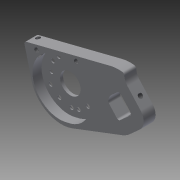
# Autodesk Inventor part: mountthatshopefullyslightlyeasiertomachine
Saved by Autodesk Inventor 2014 SP1 (Build 180222100, 222)
## iProperties
Created: 2014-05-15
Part Number: mountthatshopefullyslightlyeasiertomachine
Material: Generic
Document SubType Name: Modeling
Designer: brent
Density: 1 g/cm^3
Appearance: Default
Author: brent
Autodesk Inventor part; units mm, degrees
ref_plane "YZ Plane" through (0, 0, 0) normal (1, 0, 0) x (0, 1, 0)
ref_plane "XZ Plane" through (0, 0, 0) normal (0, 1, 0) x (-1, 0, 0)
ref_plane "XY Plane" through (0, 0, 0) normal (0, 0, 1) x (1, 0, 0)
derived "mountsketch_alt.ipt"
sketch "Sketch1" plane through (0, 0, 0) normal (0, 0, 1) x (1, 0, 0)
  circle A0 centre (-34.7277, 175.7429) radius 11 projected
  circle A1 centre (-53.3698, 187.425) radius 2.15 projected
  circle A2 centre (-34.7277, 175.7429) radius 33 projected
  circle A3 centre (-46.4099, 157.1008) radius 2.15 projected
  circle A4 centre (-16.0856, 164.0607) radius 2.15 projected
  circle A5 centre (-23.0456, 194.3849) radius 2.15 projected
  line L0 (127, 127.3759) -> (61.9125, 127.3759) projected
  line L1 (-105.8581, 0) -> (165.8097, 0) projected
  line L2 (33.0604, 216.3483) -> (58.3844, 188.2233) projected
  line L3 (58.3844, 188.2233) -> (34.6008, 166.8084) projected
  line L4 (-23.0456, 194.3849) -> (-16.0856, 164.0607) projected
  line L5 (-34.7277, 175.7429) -> (26.1158, 189.7076) projected
  line L6 (26.1158, 189.7076) -> (-32.871, 176.169) projected
  circle A6 centre (-10.8773, 175.6436) radius 2.15 projected
  line L7 (26.1158, 189.7076) -> (-36.5845, 175.3167) projected
  circle A7 centre (-25.9478, 156.059) radius 2.15 projected
  circle A8 centre (-32.3456, 198.1627) radius 2.15 projected
  circle A9 centre (-54.8647, 176.6944) radius 2.15 projected
  circle A10 centre (-33.3964, 154.1753) radius 2.15 projected
  circle A11 centre (-17.3267, 185.9534) radius 2.15 projected
  circle A12 centre (-47.2211, 194.5745) radius 2.15 projected
  circle A13 centre (-55.8422, 164.68) radius 2.15 projected
  line L8 (16.1602, 187.2887) -> (24.9131, 177.5677) projected
  line L9 (25.6305, 177.5301) -> (38.2774, 188.9173) projected
  line L10 (38.315, 189.6348) -> (29.5621, 199.3558) projected
  line L11 (33.0604, 216.3483) -> (-38.3131, 208.5475) projected
  line L12 (34.6008, 166.8084) -> (-22.9948, 144.8991) projected
  circle A14 centre (26.1158, 189.7076) radius 34.33 projected
  line L13 (33.0604, 216.3483) -> (32.281, 223.4794) projected
  line L14 (27.0217, 204.0752) -> (40.4485, 189.1632) projected
  line L15 (16.1602, 187.2887) -> (26.1028, 176.2463) projected
  line L16 (26.1028, 176.2463) -> (40.4485, 189.1632) projected
  line L17 (27.0217, 204.0752) -> (19.3412, 197.1596) projected
  ellipse E0 centre (22.8611, 193.3223) end of major axis (29.5621, 199.3558) minor radius 5.2071 (19.3412, 197.1596) -> (16.1602, 187.2887) ccw projected
  line L18 (-42.7935, 207.742) -> (17.725, 222.9963) projected
  line L19 (-42.7935, 207.742) -> (-74.7926, 199.6762) projected
  line L20 (-74.7926, 199.6762) -> (-66.7269, 167.6771) projected
  point P0 (0, 0)
  point P1 (-2.1526, 151.7421)
  point P2 (-7.3054, 194.1009)
  point P3 (0.7264, 212.8144)
  constraints: 4 other
extrude "Extrusion11" add sketch "Sketch1" along normal blind 12.7 contours A2 A14 | L11 A14 A2 | A2 L18 A14 L11 | A2 L20 L19 | A14 L11 L2 L3 L12 A2 | A2 L5 A14 | A14 L13 L11 | A2 A14 L5 | A2 A14 L12
fillet "Fillet7" radius 25.4 1 edges at (34.6008, 166.8084, 6.35)
fillet "Fillet7" radius 2.54 1 edges at (32.281, 223.4794, 6.35)
fillet "Fillet7" radius 12.7 2 edges at (58.3844, 188.2233, 6.35) (33.0604, 216.3483, 6.35)
sketch "Sketch17" plane through (-34.7277, 175.7429, 12.7) normal (0, 0, 1) x (0.4619488, 0.8869066, 0)
  circle A0 centre (10.9297, -21.199) radius 2.15 projected
  circle A1 centre (0, 0) radius 11 projected
  circle A2 centre (-13.4019, -16.88) radius 2.15 projected
  circle A3 centre (-19.5655, 13.6161) radius 2.15 projected
  circle A4 centre (10.9306, 19.7797) radius 2.15 projected
  circle A5 centre (17.0942, -10.7163) radius 2.15 projected
  circle A6 centre (-18.5134, -11.1439) radius 2.15 projected
  circle A7 centre (-8.4583, 18.2992) radius 2.15 projected
  circle A8 centre (20.9848, 8.2441) radius 2.15 projected
  circle A9 centre (21.9303, -1.7493) radius 2.15 projected
  circle A10 centre (-1.7493, -21.9303) radius 2.15 projected
  circle A11 centre (-21.9303, 1.7493) radius 2.15 projected
  circle A12 centre (1.7493, 21.9303) radius 2.15 projected
  arc A13 (-22.024, -18.7701) -> (22.024, 18.7701) centre (1.2357, -1.4499) ccw
  arc A14 (22.024, 18.7701) -> (-22.024, -18.7701) centre (-1.2357, 1.4499) ccw
  line L0 (-20.836, -20.2606) -> (-23.3073, -17.3608)
  line L1 (23.3073, 17.3608) -> (20.836, 20.2606)
  point P0 (65.9055, 28.4481)
  point P1 (29.8536, 27.856)
  point P2 (5.2355, 34.1004)
  point P3 (-139.8251, -111.9844)
  point P4 (3.0016, 34.3692)
  dimension "d178" = 58
  dimension "d179" = 58
  constraints: 8 point on circle, 4 end point, 4 tangent, 2 centre point, 2 coincident
  measures "d178" diameter of A14
  measures "d179" diameter of A13
sketch "Sketch12" plane through (49.8864, 197.6612, 12.7) normal (0.7431448, 0.6691306, 0) x (0, 0, -1)
  line L0 (12.7, 0) -> (12.7, 21.0486) projected
  line L1 (12.7, 13.589) -> (12.7, 0) projected
  line L2 (12.7, 13.589) -> (0, 13.589) projected
  line L3 (0, 0) -> (0, 13.589) projected
  line L4 (12.7, 0) -> (0, 0) projected
  circle A0 centre (6.35, 9.779) radius 2.413
  line L5 (12.7, 14.859) -> (12.7, 0) projected
  line L6 (12.7, 14.859) -> (0, 14.859) projected
  line L7 (0, 0) -> (0, 14.859) projected
  line L8 (12.7, 0) -> (0, 0) projected
  point P0 (12.7, -113.5104)
  dimension "d99" = 4.826
  dimension "d122" = 6.35
  dimension "d123" = 5.08
  constraints: 1 centre point
  measures "d99" diameter of A0
  measures "d122" distance from line of L0 A0.centre
  measures "d123" distance from line of L6 A0.centre
sketch "Sketch13" plane through (48.9464, 179.7253, 0) normal (0.6691306, -0.7431448, 0) x (0.7431448, 0.6691306, 0)
  line L0 (-14.5567, 12.7) -> (0, 12.7) projected
  line L1 (-18.034, 0) -> (0, 0) projected
  line L2 (-18.034, 0) -> (-18.034, 12.7) projected
  line L3 (0, 12.7) -> (-18.034, 12.7) projected
  line L4 (0, 0) -> (0, 12.7) projected
  circle A0 centre (-9.017, 6.35) radius 2.413
  point P0 (-156.634, 0)
  dimension "d100" = 4.826
  dimension "d101" = 9.017
  dimension "d102" = 6.35
  constraints: 1 centre point
  measures "d100" diameter of A0
  measures "d101" distance from line of A0.centre L4
  measures "d102" distance from line of A0.centre L0
extrude "Extrusion13" cut sketch "Sketch13" against normal blind 25.4 contours A0
extrude "Extrusion14" cut sketch "Sketch12" against normal blind 25.4 contours A0
thread "Thread5" size "10-32 UNF" class "2B" standard "ANSI Unified Screw Threads" full length
thread "Thread6" size "10-32 UNF" class "2B" standard "ANSI Unified Screw Threads" full length
sketch "Sketch16" plane through (-34.7277, 175.7429, 0) normal (0, 0, -1) x (-0.4619488, -0.8869066, 0)
  line L0 (-38.0971, 0.9443) -> (-44.0427, -11.275) projected
  line L1 (-44.0427, -11.275) -> (-60.259, -3.3847) projected
  line L2 (-60.259, -3.3847) -> (-54.3134, 8.8346) projected
  arc A0 (-65.8938, -45.2024) -> (-65.8938, -45.2024) centre (-77.7906, -49.6473) ccw projected
  line L3 (-58.5269, -64.9197) -> (-65.8938, -45.2024) projected
  arc A1 (-58.5269, -64.9197) -> (-42.1852, -72.3715) centre (-46.6302, -60.4747) ccw projected
  line L4 (-28.5493, -67.2767) -> (-42.1852, -72.3715) projected
  arc A2 (-28.5493, -67.2767) -> (-20.5555, -62.4595) centre (-37.4392, -43.4832) ccw projected
  line L5 (21.9355, -24.6543) -> (-20.5555, -62.4595) projected
  arc A3 (21.9355, -24.6543) -> (21.9355, 24.6543) centre (0, 0) ccw projected
  line L6 (-34.7521, 29.5687) -> (-5.2355, 34.1004) projected
  circle A4 centre (-1.7493, 21.9303) radius 2.15 projected
  circle A5 centre (21.9303, 1.7493) radius 2.15 projected
  circle A6 centre (1.7493, -21.9303) radius 2.15 projected
  circle A7 centre (-21.9303, -1.7493) radius 2.15 projected
  circle A8 centre (-20.9848, 8.2441) radius 2.15 projected
  circle A9 centre (8.4583, 18.2992) radius 2.15 projected
  circle A10 centre (18.5134, -11.1439) radius 2.15 projected
  circle A11 centre (-17.0942, -10.7163) radius 2.15 projected
  circle A12 centre (-10.9306, 19.7797) radius 2.15 projected
  circle A13 centre (19.5655, 13.6161) radius 2.15 projected
  circle A14 centre (13.4019, -16.88) radius 2.15 projected
  circle A15 centre (-10.9297, -21.199) radius 2.15 projected
  circle A16 centre (0, 0) radius 11 projected
  line L7 (-72.1881, 22.3034) -> (-62.1724, -42.9322)
  line L8 (-62.1724, -42.9322) -> (37.6257, -27.6099)
  line L9 (37.6257, -27.6099) -> (27.6099, 37.6257)
  line L10 (27.6099, 37.6257) -> (-72.1881, 22.3034)
  point P0 (-51.5181, 22.1934)
  point P1 (-5.2355, 34.1004)
  point P2 (139.8251, -111.9844)
  point P3 (-29.8536, 27.856)
  point P4 (-65.9055, 28.4481)
  point P5 (-30.9895, -27.5591)
  point P6 (-70.7348, -39.0877)
  point P7 (-3.0016, 34.3692)
  dimension "d117" = 100.9674
  dimension "d118" = 66
  constraints: 8 end point, 2 parallel, 1 perpendicular, 1 tangent, 9 other
  measures "d117" distance between parallel lines of L9 L7
  measures "d118" distance between parallel lines of L10 L8
extrude "Extrusion15" cut sketch "Sketch17" against normal blind 9.525 contours A14 A13
fillet "Fillet8" radius 2.3813 3 edges at (27.0217, 204.0752, 6.35) (40.4485, 189.1632, 6.35) (26.1028, 176.2463, 6.35)
fillet "Fillet9" radius 2.54 1 edges at (-74.7926, 199.6762, 6.35)
sketch "Sketch18" plane through (-34.7277, 175.7429, 0) normal (0, 0, -1) x (-0.4619488, -0.8869066, 0)
  arc A0 (-58.5269, -64.9197) -> (-42.1852, -72.3715) centre (-46.6302, -60.4747) ccw projected
  line L0 (-28.5493, -67.2767) -> (-42.1852, -72.3715) projected
  arc A1 (-28.5493, -67.2767) -> (-20.5555, -62.4595) centre (-37.4392, -43.4832) ccw projected
  line L1 (21.9355, -24.6543) -> (-20.5555, -62.4595) projected
  arc A2 (21.9355, -24.6543) -> (21.9355, 24.6543) centre (0, 0) ccw projected
  line L2 (-34.7521, 29.5687) -> (-5.2355, 34.1004) projected
  arc A3 (-41.8032, 30.5011) -> (-34.7521, 29.5687) centre (-36.6794, 42.1216) ccw projected
  arc A4 (-66.1399, -24.692) -> (-72.6369, -35.4594) centre (-40.492, -47.5116) ccw projected
  arc A5 (-72.6369, -35.4594) -> (-71.6697, -38.463) centre (-70.2585, -36.3511) ccw projected
  line L3 (-70.7348, -39.0877) -> (-71.6697, -38.463) projected
  arc A6 (-65.8938, -45.2024) -> (-65.8938, -45.2024) centre (-77.7906, -49.6473) ccw projected
  line L4 (-58.5269, -64.9197) -> (-65.8938, -45.2024) projected
  circle A7 centre (-1.7493, 21.9303) radius 2.15 projected
  circle A8 centre (21.9303, 1.7493) radius 2.15 projected
  circle A9 centre (1.7493, -21.9303) radius 2.15 projected
  circle A10 centre (-21.9303, -1.7493) radius 2.15 projected
  circle A11 centre (-20.9848, 8.2441) radius 2.15 projected
  circle A12 centre (8.4583, 18.2992) radius 2.15 projected
  circle A13 centre (18.5134, -11.1439) radius 2.15 projected
  circle A14 centre (-17.0942, -10.7163) radius 2.15 projected
  circle A15 centre (-10.9306, 19.7797) radius 2.15 projected
  circle A16 centre (19.5655, 13.6161) radius 2.15 projected
  circle A17 centre (13.4019, -16.88) radius 2.15 projected
  circle A18 centre (0, 0) radius 11 projected
  circle A19 centre (-10.9297, -21.199) radius 2.15 projected
  ellipse E0 centre (-42.1944, -42.9551) end of major axis (-50.6411, -46.111) minor radius 5.2071 (-33.7477, -39.7992) -> (-43.9717, -38.0606) ccw projected
  line L5 (-33.7477, -39.7992) -> (-29.3806, -51.4878) projected
  arc A20 (-30.7778, -54.5518) -> (-29.3806, -51.4878) centre (-31.6112, -52.3212) ccw projected
  line L6 (-30.7778, -54.5518) -> (-44.3995, -59.6413) projected
  arc A21 (-47.4636, -58.2441) -> (-44.3995, -59.6413) centre (-45.233, -57.4107) ccw projected
  line L7 (-47.4636, -58.2441) -> (-52.8198, -43.9085) projected
  arc A22 (-51.4226, -40.8445) -> (-52.8198, -43.9085) centre (-50.5891, -43.0751) ccw projected
  line L8 (-51.4226, -40.8445) -> (-43.9717, -38.0606) projected
  line L9 (-87.4828, -33.6647) -> (-43.6118, -82.9733)
  line L10 (-43.6118, -82.9733) -> (46.5898, -2.7188)
  line L11 (46.5898, -2.7188) -> (2.7188, 46.5898)
  line L12 (2.7188, 46.5898) -> (-87.4828, -33.6647)
  point P0 (139.8251, -111.9844)
  point P1 (-65.4837, -33.2012)
  point P2 (-3.0016, 34.3692)
  dimension "d125" = 66
  dimension "d126" = 120.7357
  constraints: 8 end point, 2 parallel, 1 collinear, 1 perpendicular, 1 tangent, 8 other
  measures "d125" distance between parallel lines of L10 L12
  measures "d126" distance between parallel lines of L11 L9
sketch "Sketch19" plane through (-34.7277, 175.7429, 0) normal (0, 0, -1) x (-0.8869066, 0.4619488, 0)
  arc A0 (44.9014, 0.8211) -> (44.6922, 4.4071) centre (43.0038, 2.5095) ccw projected
  line L0 (-24.692, 66.1399) -> (44.6922, 4.4071) projected
  arc A1 (-24.692, 66.1399) -> (-35.4594, 72.6369) centre (-47.5116, 40.492) ccw projected
  arc A2 (-35.4594, 72.6369) -> (-38.463, 71.6697) centre (-36.3511, 70.2585) ccw projected
  arc A3 (-45.2024, 65.8938) -> (-45.2024, 65.8938) centre (-49.6473, 77.7906) ccw projected
  line L1 (-64.9197, 58.5269) -> (-45.2024, 65.8938) projected
  arc A4 (-64.9197, 58.5269) -> (-72.3715, 42.1852) centre (-60.4747, 46.6302) ccw projected
  line L2 (-67.2767, 28.5493) -> (-72.3715, 42.1852) projected
  arc A5 (-67.2767, 28.5493) -> (-62.4595, 20.5555) centre (-43.4832, 37.4392) ccw projected
  line L3 (-24.6543, -21.9355) -> (-62.4595, 20.5555) projected
  arc A6 (-24.6543, -21.9355) -> (24.6543, -21.9355) centre (0, 0) ccw projected
  line L4 (44.9014, 0.8211) -> (24.6543, -21.9355) projected
  ellipse E0 centre (-42.9551, 42.1944) end of major axis (-46.111, 50.6411) minor radius 5.2071 (-39.7992, 33.7477) -> (-38.0606, 43.9717) ccw projected
  line L5 (-39.7992, 33.7477) -> (-51.4878, 29.3806) projected
  arc A7 (-54.5518, 30.7778) -> (-51.4878, 29.3806) centre (-52.3212, 31.6112) ccw projected
  line L6 (-54.5518, 30.7778) -> (-59.6413, 44.3995) projected
  arc A8 (-58.2441, 47.4636) -> (-59.6413, 44.3995) centre (-57.4107, 45.233) ccw projected
  line L7 (-58.2441, 47.4636) -> (-43.9085, 52.8198) projected
  arc A9 (-40.8445, 51.4226) -> (-43.9085, 52.8198) centre (-43.0751, 50.5891) ccw projected
  line L8 (-40.8445, 51.4226) -> (-38.0606, 43.9717) projected
  circle A10 centre (0, 0) radius 11 projected
  circle A11 centre (-21.199, 10.9297) radius 2.15 projected
  circle A12 centre (-16.88, -13.4019) radius 2.15 projected
  circle A13 centre (13.6161, -19.5655) radius 2.15 projected
  circle A14 centre (19.7797, 10.9306) radius 2.15 projected
  circle A15 centre (-10.7163, 17.0942) radius 2.15 projected
  circle A16 centre (-11.1439, -18.5134) radius 2.15 projected
  circle A17 centre (18.2992, -8.4583) radius 2.15 projected
  circle A18 centre (8.2441, 20.9848) radius 2.15 projected
  circle A19 centre (-1.7493, 21.9303) radius 2.15 projected
  circle A20 centre (-21.9303, -1.7493) radius 2.15 projected
  circle A21 centre (1.7493, -21.9303) radius 2.15 projected
  circle A22 centre (21.9303, 1.7493) radius 2.15 projected
  line L9 (-88.3349, 34.4229) -> (-44.4639, 83.7315)
  line L10 (-44.4639, 83.7315) -> (46.5898, 2.7188)
  line L11 (46.5898, 2.7188) -> (2.7188, -46.5898)
  line L12 (2.7188, -46.5898) -> (-88.3349, 34.4229)
  point P0 (-33.2012, 65.4837)
  point P1 (-111.9844, -139.8251)
  dimension "d128" = 66
  dimension "d129" = 121.8763
  constraints: 8 end point, 3 tangent, 2 parallel, 1 collinear, 1 perpendicular, 1 point on line, 3 other
  measures "d128" distance between parallel lines of L12 L10
  measures "d129" distance between parallel lines of L11 L9
sketch "Sketch21" plane through (17.725, 222.9963, 12.7) normal (-0.2444163, 0.9696704, 0) x (0.9696704, 0.2444163, 0)
  line L0 (0, 12.7) -> (-92.8714, 12.7) projected
  circle A0 centre (-89.0614, 8.89) radius 2.413
  line L1 (-95.4114, 12.7) -> (-95.4114, 0) projected
  point P0 (-71.6914, 12.7)
  dimension "d138" = 4.826
  dimension "d140" = 3.81
  dimension "d167" = 6.35
  constraints: 1 centre point
  measures "d138" diameter of A0
  measures "d140" distance from line of A0.centre L0
  measures "d167" distance from line of L1 A0.centre
extrude "Extrusion17" cut sketch "Sketch21" against normal blind 12.7
thread "Thread7" size "10-32 UNF" class "2B" standard "ANSI Unified Screw Threads" full length
sketch "Sketch22" plane through (-34.7277, 175.7429, 0) normal (0, 0, -1) x (-0.8869066, 0.4619488, 0)
  arc A0 (-24.692, 66.1399) -> (-35.4594, 72.6369) centre (-47.5116, 40.492) ccw projected
  circle A1 centre (0, 0) radius 11 projected
  circle A2 centre (-47.5116, 40.492) radius 31.83
  circle A3 centre (0, 0) radius 11.935
  line L0 (10.2328, 6.1427) -> (-20.2212, 56.8743)
  line L1 (-59.3607, 10.9497) -> (-4.4429, -11.0772)
  circle A4 centre (0, 0) radius 28
  circle A5 centre (1.2967, 36.6425) radius 2.413
  circle A6 centre (33.9359, 7.6026) radius 2.413
  line L2 (0, 0) -> (-47.5116, 40.492)
  line L3 (-24.692, 66.1399) -> (44.6922, 4.4071) projected
  line L4 (44.9014, 0.8211) -> (24.6543, -21.9355) projected
  point P0 (-111.9844, -139.8251)
  dimension "d146" = 63.66
  dimension "d147" = 23.87
  dimension "d148" = 56
  dimension "d149" = 4.826
  dimension "d150" = 4.826
  dimension "d181" = 12.7
  dimension "d182" = 4.7625
  dimension "d184" = 4.7625
  dimension "d185" = 43.688
  constraints: 6 end point, 5 centre point, 4 point on circle, 4 tangent, 3 coincident
  measures "d146" diameter of A2
  measures "d147" diameter of A3
  measures "d148" diameter of A4
  measures "d149" diameter of A5
  measures "d150" diameter of A6
  measures "d181" distance from line of L4 A6.centre
  measures "d182" distance from line of L3 A6.centre
  measures "d184" distance from line of L3 A5.centre
  measures "d185" distance of A6.centre A5.centre
extrude "Extrusion18" cut sketch "Sketch22" against normal through all contours A5 | A6
chamfer "Chamfer1" distance 2.2 angle 45 12 edges at (-34.4956, 198.1627, 0) (-49.3711, 194.5745, 0) (-55.5198, 187.425, 0) (-57.0147, 176.6944, 0) (-57.9922, 164.68, 0) (-48.5599, 157.1008, 0) (-35.5464, 154.1753, 0) (-28.0978, 156.059, 0) (-18.2356, 164.0607, 0) (-13.0273, 175.6436, 0) (-19.4767, 185.9534, 0) (-25.1956, 194.3849, 0)
thread "Thread12" size "10-32 UNF" class "2B" standard "ANSI Unified Screw Threads" full length
thread "Thread13" size "10-32 UNF" class "2B" standard "ANSI Unified Screw Threads" full length
sketch "Sketch26" plane through (-66.7269, 167.6771, 0) normal (-0.9696704, -0.2444163, 0) x (0, 0, 1)
  line L0 (12.7, 30.46) -> (12.7, 0) projected
  line L1 (1.397, 33) -> (6.223, 33) projected
  line L2 (12.7, 30.6505) -> (12.7, 25.8245) projected
  line L3 (0, 25.8245) -> (12.7, 25.8245) projected
  line L4 (0, 30.6505) -> (12.7, 30.6505) projected
  circle A0 centre (8.89, 22.0145) radius 2.413
  point P0 (0, -178.9007)
  dimension "d192" = 4.826
  dimension "d193" = 3.81
  dimension "d194" = 3.81
  constraints: 1 centre point
  measures "d192" diameter of A0
  measures "d193" distance from line of L0 A0.centre
  measures "d194" distance from line of A0.centre L3
extrude "Extrusion21" cut sketch "Sketch26" against normal blind 25.4
thread "Thread14" size "10-32 UNF" class "2B" standard "ANSI Unified Screw Threads" full length
equation "\"d91\" = mount_thickness"
equation "\"d120\" = mount_thickness - mount_motor_thickness"
equation "\"mount_thickness\" = 12.7"
equation "\"mount_motor_thickness\" = 3.175"
body "Solid1"
body "Solid3"
